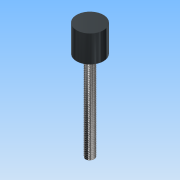
# Autodesk Inventor part: регулировочный  винт  концевика
Saved by Autodesk Inventor 2017 (Build 210142000, 142)
## iProperties
Part Number: регулировочный  винт  концевика
Material: Типовые
Document SubType Name: Modeling
Designer: Max
Mass: 1.74204 g
Surface Area: 22.4025 cm^2
Volume: 1.74204 cm^3
Density: 1 g/cm^3
Appearance: Сталь — полированная
Author: Max
Autodesk Inventor part; units mm, degrees
ref_plane "YZ Plane" through (0, 0, 0) normal (1, 0, 0) x (0, 1, 0)
ref_plane "XZ Plane" through (0, 0, 0) normal (0, 1, 0) x (-1, 0, 0)
ref_plane "XY Plane" through (0, 0, 0) normal (0, 0, 1) x (1, 0, 0)
sketch "Эскиз1" plane through (0, 0, 0) normal (0, 0, 1) x (1, 0, 0)
  circle A0 centre (0, 0) radius 6
  circle A1 centre (0, 0) radius 2
  dimension "d0" = 12
  dimension "d1" = 4
  constraints: 2 centre point, 2 coincident
  measures "d0" diameter of A0
  measures "d1" diameter of A1
extrude "Выдавливание1" add sketch "Эскиз1" along normal blind 12 contours A0 | A1
extrude "Выдавливание2" add sketch "Эскиз1" against normal blind 40 contours A1
thread "Резьба1" size "M4x0.7" class "6g" standard "ANSI Metric M Profile" full length
sketch "Эскиз3" plane through (0, 0, -40) normal (1, 0, 0) x (0, 1, 0)
  line L0 (2, 0) -> (2, 40)
  line L1 (2, 40) -> (1.481, 40)
  line L2 (1.481, 40) -> (1.481, 0)
  line L3 (1.481, 0) -> (2, 0)
  line L4 (0, -11.3161) -> (0, 62.5527) projected
  constraints: 8 end point
revolve "Вращение1" cut sketch "Эскиз3" angle 360 about axis through (0, 0, -40) along (0, 0, 1)
sketch "Эскиз4" plane through (0, 0, -40) normal (1, 0, 0) x (0, 1, 0)
  line L0 (2, 0) -> (2, 40)
  line L1 (2, 40) -> (1.481, 40)
  line L2 (1.481, 40) -> (1.481, 0)
  line L3 (1.481, 0) -> (2, 0)
  line L4 (0, -11.3161) -> (0, 62.5527) projected
  constraints: 8 end point
revolve "Вращение2" add sketch "Эскиз4" angle 360 about axis through (0, 0, -40) along (0, 0, 1) separate body
sketch "Эскиз2" plane through (0, 0, -40) normal (-1, 0, 0) x (0, 0, 1)
  line L0 (-0.4084, -1.5165) -> (-0.3501, -1.5165) construction
  line L1 (0.0582, -1.9648) -> (-0.0001, -2.0768) construction
  line L2 (-0.7001, -2.0768) -> (-0.7584, -1.9648) construction
  line L3 (-0.2918, -1.5165) -> (-0.3501, -1.4045) construction
  line L4 (-0.3501, -1.4045) -> (-0.4084, -1.5165) construction
  line L5 (-0.7001, -2.0768) -> (-0.6418, -1.9648) construction
  line L6 (-0.2918, -1.5165) -> (-0.0584, -1.9648)
  line L7 (-0.7584, -1.9648) -> (-0.6418, -1.9648) construction
  arc A0 (-0.7584, -1.9648) -> (-0.7001, -2.0002) centre (-0.7001, -1.9344) ccw construction
  line L8 (0.0582, -1.9648) -> (-0.0584, -1.9648) construction
  line L9 (-0.7001, -2.0768) -> (-0.7001, -1.9648) construction
  line L10 (-0.0001, -2.0768) -> (-0.0001, -1.9648) construction
  line L11 (-0.3501, -1.4045) -> (-0.3501, -1.4811) construction
  line L12 (-0.7001, -2.0002) -> (-0.0001, -2.0002)
  arc A1 (-0.7001, -2.0002) -> (-0.6418, -1.9648) centre (-0.7001, -1.9344) ccw
  line L13 (-0.0584, -1.9648) -> (-0.0001, -2.0768) construction
  line L14 (-0.6418, -1.9648) -> (-0.4084, -1.5165)
  line L15 (-0.0001, -0.0002) -> (-0.0001, 0.0177)
  line L16 (-0.0001, 0.0177) -> (-0.0001, -0.0002)
  line L17 (-0.0001, -0.0002) -> (0.0334, -0.0002)
  arc A2 (-0.0584, -1.9648) -> (-0.0001, -2.0002) centre (-0.0001, -1.9344) ccw
  arc A3 (-0.0001, -2.0002) -> (0.0582, -1.9648) centre (-0.0001, -1.9344) ccw construction
  arc A4 (-0.3501, -1.4811) -> (-0.4084, -1.5165) centre (-0.3501, -1.5469) ccw
  arc A5 (-0.2918, -1.5165) -> (-0.3501, -1.4811) centre (-0.3501, -1.5469) ccw
  line L18 (-0.3501, -1.4811) -> (-0.3501, -1.5165) construction
  line L19 (-0.3501, -1.5165) -> (-0.2918, -1.5165) construction
  dimension "d8" = 55
  dimension "d9" = 0.1121
  dimension "d10" = 0.1121
  dimension "Эскиз2_ThreadOffset" = 0
  dimension "Эскиз2_MajorRadius" = 2
  dimension "d13" = 0.7
  dimension "Эскиз2_MinorRadius" = 1.481
  constraints: 40 end point, 12 point on circle, 10 parallel, 8 tangent, 6 centre point, 6 collinear, 2 midpoint, 2 point on line, 1 horizontal, 1 perpendicular, 3 other
  measures "d8" angle of L6 L14
  measures "d9" distance of L3.end L0.end
  measures "d10" distance of L1.end L10.end
  measures "Эскиз2_ThreadOffset" distance between parallel lines of L15 L10
  measures "Эскиз2_MajorRadius" distance from line of L12 L15.start
  measures "d13" distance from line of L1.end L9
  measures "Эскиз2_MinorRadius" distance edge to line of A5 L17
coil "Пружина1" sketch "Эскиз2" operation cut axis through (0, 0, -40) along (0, 0, 1) pitch 0.7007 turns 59.083773 hand right bodies 2
equation "\"d8\" = d15"
equation "\"d9\" = 0.160083 * Эскиз2_Pitch"
equation "\"d10\" = 0.160083 * Эскиз2_Pitch"
equation "\"d13\" = Эскиз2_Pitch"
equation "\"d15\" = 55deg"
equation "\"Эскиз2_Pitch\" = 0.7"
